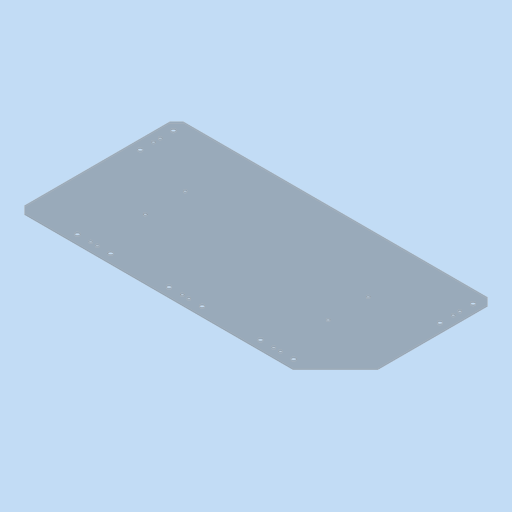
# Autodesk Inventor part: enc-SidePanel 357x708
Saved by Autodesk Inventor 2023.2 (Build 272271000, 271)
## iProperties
Created: 2023-11-30
Part Number: enc-SidePanel 357x708
Material: Generisch
Document SubType Name: Modeling
Designer: Nils Bade
Density: 1 g/cm^3
Appearance: PVC Verglasung
Author: Nils Bade
Autodesk Inventor part; units mm, degrees
ref_plane "YZ Plane" through (0, 0, 0) normal (1, 0, 0) x (0, 1, 0)
ref_plane "XZ Plane" through (0, 0, 0) normal (0, 1, 0) x (-1, 0, 0)
ref_plane "XY Plane" through (0, 0, 0) normal (0, 0, 1) x (1, 0, 0)
sketch "Skizze1" plane through (0, 0, 0) normal (0, 1, 0) x (-1, 0, 0)
  line L0 (0, 0) -> (-708, 0)
  line L1 (-708, 0) -> (-708, 357)
  line L2 (-708, 357) -> (0, 357)
  line L3 (0, 357) -> (0, 0)
  line L4 (-354, 0) -> (-354, 357) construction
  line L5 (0, 178.5) -> (-708, 178.5) construction
  line L6 (-150, 0) -> (-150, 357) construction
  line L7 (-558, 0) -> (-558, 357) construction
  line L8 (-708, 67) -> (0, 67) construction
  line L9 (0, 71.4) -> (-708, 71.4) construction
  line L10 (-688, 337) -> (-688, 20) construction
  line L11 (-688, 20) -> (-20, 20) construction
  line L12 (-20, 20) -> (-20, 337) construction
  line L13 (-20, 337) -> (-688, 337) construction
  line L14 (-28, 19.5) -> (-12, 19.5) construction
  line L15 (-12, 19.5) -> (-12, 114.5) construction
  line L16 (-12, 114.5) -> (-28, 114.5) construction
  line L17 (-28, 114.5) -> (-28, 19.5) construction
  line L18 (-28, 19.5) -> (-12, 114.5) construction
  line L19 (-12, 19.5) -> (-28, 114.5) construction
  line L20 (-102.5, 345) -> (-197.5, 345) construction
  line L21 (-197.5, 345) -> (-197.5, 329) construction
  line L22 (-197.5, 329) -> (-102.5, 329) construction
  line L23 (-102.5, 329) -> (-102.5, 345) construction
  line L24 (-102.5, 345) -> (-197.5, 329) construction
  line L25 (-197.5, 345) -> (-102.5, 329) construction
  line L26 (-306.5, 345) -> (-401.5, 345) construction
  line L27 (-401.5, 345) -> (-401.5, 329) construction
  line L28 (-401.5, 329) -> (-306.5, 329) construction
  line L29 (-306.5, 329) -> (-306.5, 345) construction
  line L30 (-306.5, 345) -> (-401.5, 329) construction
  line L31 (-401.5, 345) -> (-306.5, 329) construction
  circle A0 centre (-20, 59.5) radius 3.25
  circle A1 centre (-20, 30) radius 4.5
  circle A2 centre (-20, 74.5) radius 3.25
  circle A3 centre (-20, 104) radius 4.5
  circle A4 centre (-142.5, 337) radius 3.25
  circle A5 centre (-113, 337) radius 4.5
  circle A6 centre (-317, 337) radius 4.5
  circle A7 centre (-346.5, 337) radius 3.25
  circle A8 centre (-157.5, 337) radius 3.25
  circle A9 centre (-187, 337) radius 4.5
  circle A10 centre (-391, 337) radius 4.5
  circle A11 centre (-361.5, 337) radius 3.25
  circle A12 centre (-688, 59.5) radius 3.25
  circle A13 centre (-688, 30) radius 4.5
  circle A14 centre (-688, 104) radius 4.5
  circle A15 centre (-688, 74.5) radius 3.25
  circle A16 centre (-565.5, 337) radius 3.25
  circle A17 centre (-595, 337) radius 4.5
  circle A18 centre (-550.5, 337) radius 3.25
  circle A19 centre (-521, 337) radius 4.5
  circle A20 centre (-150, 134) radius 3.25
  line L32 (-138.5, 124.5) -> (-161.5, 124.5) construction
  line L33 (-161.5, 124.5) -> (-161.5, 232.5) construction
  line L34 (-161.5, 232.5) -> (-138.5, 232.5) construction
  line L35 (-138.5, 232.5) -> (-138.5, 124.5) construction
  line L36 (-138.5, 124.5) -> (-161.5, 232.5) construction
  line L37 (-161.5, 124.5) -> (-138.5, 232.5) construction
  circle A21 centre (-150, 223) radius 3.25
  circle A22 centre (-558, 134) radius 3.25
  circle A23 centre (-558, 223) radius 3.25
  line L38 (-857.6188, 167) -> (175.5187, 167) construction
  line L39 (-857.6403, 142) -> (175.5402, 142) construction
  line L40 (-708, 317) -> (0, 317) construction
  line L41 (-668, 357) -> (-668, 0) construction
  line L42 (-708, 262) -> (-599.5, 262) construction
  line L43 (-613, 357) -> (-613, 217.4879) construction
  line L44 (-613, 357) -> (-708, 262)
  line L45 (-708, 3) -> (0, 3)
  point P0 (-20, 67)
  point P1 (-150, 337)
  point P2 (-354, 337)
  point P3 (-150, 178.5)
  dimension "d0" = 708
  dimension "d1" = 357
  dimension "d2" = 290
  dimension "d3" = 71.4
  dimension "d4" = 150
  dimension "d5" = 150
  dimension "d6" = 20
  dimension "d7" = 16
  dimension "d8" = 95
  dimension "d9" = 95
  dimension "d10" = 16
  dimension "d11" = 95
  dimension "d12" = 16
  dimension "d13" = 6.5
  dimension "d14" = 7.5
  dimension "d15" = 9
  dimension "d16" = 37
  dimension "d17" = 6.5
  dimension "d18" = 9
  dimension "d19" = 7.5
  dimension "d20" = 37
  dimension "d21" = 6.5
  dimension "d22" = 9
  dimension "d23" = 7.5
  dimension "d24" = 37
  dimension "d30" = 6.5
  dimension "d31" = 44.5
  dimension "d32" = 23
  dimension "d33" = 108
  dimension "d34" = 190
  dimension "d35" = 25
  dimension "d36" = 40
  dimension "d37" = 40
  dimension "d47" = 95
  dimension "d48" = 95
  dimension "d49" = 3
  constraints: 92 end point, 27 point on line, 24 centre point, 17 symmetric about line, 14 midpoint, 13 parallel, 13 perpendicular, 7 horizontal, 1 vertical, 20 other
  measures "d0" distance of L0.start L0.end
  measures "d1" distance of L2.end L0.start
  measures "d2" distance between parallel lines of L2 L8
  measures "d3" distance between parallel lines of L0 L9
  measures "d4" distance between parallel lines of L3 L6
  measures "d5" distance between parallel lines of L1 L7
  measures "d6" distance between parallel lines of L1 L10
  measures "d7" distance of L16.end L15.end
  measures "d8" distance of L15.end L14.end
  measures "d9" distance of L22.end L21.end
  measures "d10" distance of L21.end L20.end
  measures "d11" distance of L28.end L27.end
  measures "d12" distance of L27.end L26.end
  measures "d13" diameter of A0
  measures "d14" distance from line of L8 A0.centre
  measures "d15" diameter of A1
  measures "d16" distance from line of L8 A1.centre
  measures "d17" diameter of A4
  measures "d18" diameter of A5
  measures "d19" distance from line of L6 A4.centre
  measures "d20" distance from line of L6 A5.centre
  measures "d21" diameter of A7
  measures "d22" diameter of A6
  measures "d23" distance from line of L4 A7.centre
  measures "d24" distance from line of L4 A6.centre
  measures "d30" diameter of A20
  measures "d31" distance from line of L5 A20.centre
  measures "d32" distance of L33.end L34.end
  measures "d33" distance of L32.end L33.end
  measures "d34" distance between parallel lines of L2 L38
  measures "d35" distance between parallel lines of L39 L38
  measures "d36" distance between parallel lines of L2 L40
  measures "d37" distance between parallel lines of L1 L41
  measures "d47" distance between parallel lines of L2 L42
  measures "d48" distance between parallel lines of L1 L43
  measures "d49" distance between parallel lines of L0 L45
extrude "Ex1 mit Z-untermaß" add sketch "Skizze1" along normal blind 3 contours L45 L1 L44 L2 L3
chamfer "Fase1" distance 15 angle 45 3 edges at (0, 1.5, 357) (0, 1.5, 3) (708, 1.5, 3)
equation "\"d3\" = 0.2 * d1"
equation "\"d5\" = d4"
equation "\"d17\" = d13"
equation "\"d18\" = d15"
equation "\"d19\" = d14"
equation "\"d20\" = d16"
equation "\"d21\" = d13"
equation "\"d22\" = d15"
equation "\"d23\" = d14"
equation "\"d24\" = d16"
